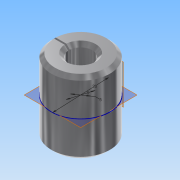
# Autodesk Inventor part: муфта
Saved by Autodesk Inventor 2017 (Build 210142000, 142)
## iProperties
Part Number: муфта
Material: Типовые
Document SubType Name: Modeling
Designer: Max
Density: 1 g/cm^3
Appearance: Алюминий — темный
Mass: 6.61019 g
Surface Area: 33.4899 cm^2
Volume: 6.61019 cm^3
Author: Max
Autodesk Inventor part; units mm, degrees
ref_plane "YZ Plane" through (0, 0, 0) normal (1, 0, 0) x (0, 1, 0)
ref_plane "XZ Plane" through (0, 0, 0) normal (0, 1, 0) x (-1, 0, 0)
ref_plane "XY Plane" through (0, 0, 0) normal (0, 0, 1) x (1, 0, 0)
sketch "Эскиз1" plane through (0, 0, 0) normal (0, 0, 1) x (1, 0, 0)
  circle A0 centre (0, 0) radius 10
  circle A1 centre (0, 0) radius 4
  circle A2 centre (0, 0) radius 2.5
  dimension "d0" = 20
  dimension "d1" = 8
  dimension "d2" = 5
  constraints: 3 centre point, 3 coincident
  measures "d0" diameter of A0
  measures "d1" diameter of A1
  measures "d2" diameter of A2
extrude "Выдавливание1" add sketch "Эскиз1" along normal blind 12.5 contours A0
extrude "Выдавливание2" add sketch "Эскиз1" against normal blind 12.5 contours A0 | A1
chamfer "Фаска1" distance 1.2 angle 45 4 edges at (-10, 0, -12.5) (-10, 0, 12.5) (-2.5, 0, -12.5) (-4, 0, 12.5)
sketch "Эскиз2" plane through (0, 0, -12.5) normal (0, 0, -1) x (-1, 0, 0)
  line L0 (10.8628, -0.3) -> (-0.9121, -0.3)
  line L1 (-0.9121, -0.3) -> (-0.9121, 0.3)
  line L2 (-0.9121, 0.3) -> (10.8628, 0.3)
  line L3 (10.8628, 0.3) -> (10.8628, -0.3)
  line L4 (10.8628, -0.3) -> (-0.9121, 0.3) construction
  line L5 (-0.9121, -0.3) -> (10.8628, 0.3) construction
  point P0 (0, 0)
  point P1 (4.9754, 0)
  dimension "d10" = 0.6
  dimension "d11" = 4.9754
  constraints: 12 end point, 2 midpoint, 2 parallel, 1 horizontal, 1 perpendicular
  measures "d10" distance between parallel lines of L0 L2
  measures "d11" distance of point (0, 0) point (4.975, 0)
extrude "Выдавливание3" cut sketch "Эскиз2" against normal blind 30
ref_plane "РабПлоскость1" through (0, 0, 0) normal (0, 0, -1) x (-1, 0, 0)
sketch "Эскиз3" plane through (0, 0, 0) normal (0, 0, -1) x (-1, 0, 0)
  circle A0 centre (0, 0) radius 10
  arc A1 (9.9955, 0.3) -> (9.9955, -0.3) centre (0, 0) ccw projected
  line L0 (-9.9999, -0.037) -> (9.9999, -0.037)
  constraints: 3 point on circle, 2 end point, 1 centre point, 1 coincident, 1 horizontal
extrude "Выдавливание4" cut sketch "Эскиз3" along normal mid plane 0.6 contours A0 L0 picked at (0.3426, 3.291)
sketch "Эскиз4" plane through (-8.7949, -0.3, -12.5) normal (0, 1, 0) x (1, 0, 0)
  circle A0 centre (1.7949, -6.25) radius 1.5
  circle A1 centre (1.7949, -18.75) radius 1.5
  line L0 (0, 0) -> (17.5949, 0) projected
  line L1 (17.5949, -25) -> (0, -25) projected
  point P0 (8.7949, -12.5)
  dimension "d17" = 3
  dimension "d18" = 3
  dimension "d19" = 6.25
  dimension "d20" = 6.25
  dimension "d21" = 7
  dimension "d22" = 7
  constraints: 2 centre point
  measures "d17" diameter of A0
  measures "d18" diameter of A1
  measures "d19" distance from line of L0 A0.centre
  measures "d20" distance from line of L1 A1.centre
  measures "d21" horizontal distance of point (8.795, -12.5) A0.centre
  measures "d22" horizontal distance of point (8.795, -12.5) A1.centre
extrude "Выдавливание5" cut sketch "Эскиз4" along normal blind 20
ref_plane "РабПлоскость2" through (-8.7949, 16.8, -12.5) normal (0, -1, 0) x (1, 0, 0)
sketch "Эскиз5" plane through (-8.7949, 16.8, -12.5) normal (0, -1, 0) x (1, 0, 0)
  spline S0 degree 4 poles (3.2949, 6.25) (3.2949, 5.9602) (3.2208, 5.6699) (3.0692, 5.4082) (2.6878, 5.0172) (2.4668, 4.8772) (2.2335, 4.7973) (1.7464, 4.728) (1.4956, 4.754) (1.2664, 4.8269) (0.9398, 5.0096) (0.8262, 5.0933) (0.7218, 5.1917) (0.5611, 5.39) (0.4993, 5.4829) (0.4449, 5.5852) (0.3514, 5.8208) (0.3144, 5.9563) (0.2949, 6.1031) (0.2949, 6.3424) (0.3027, 6.4345) (0.3175, 6.5243) (0.3688, 6.7319) (0.4112, 6.8451) (0.4631, 6.9492) (0.628, 7.2136) (0.7581, 7.3549) (0.9035, 7.4706) (1.203, 7.6372) (1.3518, 7.6953) (1.5105, 7.7323) (1.8327, 7.7576) (1.9958, 7.7485) (2.1612, 7.7149) (2.4707, 7.5983) (2.6146, 7.5207) (2.7487, 7.4198) (3.0679, 7.0941) (3.2204, 6.8318) (3.2949, 6.5407) (3.2949, 6.25) knots 0 0 0 0 0 0.110553 0.110553 0.110553 0.210117 0.210117 0.210117 0.323911 0.323911 0.323911 0.392633 0.392633 0.392633 0.443405 0.443405 0.443405 0.499546 0.499546 0.499546 0.534863 0.534863 0.534863 0.585287 0.585287 0.585287 0.6758 0.6758 0.6758 0.752528 0.752528 0.752528 0.824124 0.824124 0.824124 0.888854 0.888854 0.888854 1 1 1 1 1 projected
  spline S1 degree 4 poles (3.2949, 18.75) (3.2949, 18.4602) (3.2208, 18.1699) (3.0692, 17.9082) (2.6878, 17.5172) (2.4668, 17.3772) (2.2335, 17.2973) (1.7464, 17.228) (1.4956, 17.254) (1.2664, 17.3269) (0.9398, 17.5096) (0.8262, 17.5933) (0.7218, 17.6917) (0.5611, 17.89) (0.4993, 17.9829) (0.4449, 18.0852) (0.3514, 18.3208) (0.3144, 18.4563) (0.2949, 18.6031) (0.2949, 18.8424) (0.3027, 18.9345) (0.3175, 19.0243) (0.3688, 19.2319) (0.4112, 19.3451) (0.4631, 19.4492) (0.628, 19.7136) (0.7581, 19.8549) (0.9035, 19.9706) (1.203, 20.1372) (1.3518, 20.1953) (1.5105, 20.2323) (1.8327, 20.2576) (1.9958, 20.2485) (2.1612, 20.2149) (2.4707, 20.0983) (2.6146, 20.0207) (2.7487, 19.9198) (3.0679, 19.5941) (3.2204, 19.3318) (3.2949, 19.0407) (3.2949, 18.75) knots 0 0 0 0 0 0.110553 0.110553 0.110553 0.210117 0.210117 0.210117 0.323911 0.323911 0.323911 0.392633 0.392633 0.392633 0.443405 0.443405 0.443405 0.499546 0.499546 0.499546 0.534863 0.534863 0.534863 0.585287 0.585287 0.585287 0.6758 0.6758 0.6758 0.752528 0.752528 0.752528 0.824124 0.824124 0.824124 0.888854 0.888854 0.888854 1 1 1 1 1 projected
  circle A0 centre (1.7949, 6.25) radius 1.5 projected
  circle A1 centre (1.7949, 6.25) radius 2.25
  circle A2 centre (1.7949, 18.75) radius 1.5 projected
  circle A3 centre (1.7949, 18.75) radius 2.25
  point P0 (8.7949, 12.5)
  dimension "d26" = 4.5
  dimension "d27" = 4.5
  constraints: 2 centre point, 2 coincident, 2 horizontal alignment, 2 other
  measures "d26" diameter of A1
  measures "d27" diameter of A3
extrude "Выдавливание6" cut sketch "Эскиз5" along normal blind 14 contours S0 | S1 | A1 | A3
sketch "Эскиз6" plane through (-7, 2.8, -6.25) normal (0, 1, 0) x (1, 0, 0)
  circle A0 centre (0, 0) radius 1.5 projected
  circle A1 centre (0, 0) radius 2.25 projected
  circle A2 centre (0, -12.5) radius 1.5 projected
  circle A3 centre (0, -12.5) radius 2.25 projected
  circle A4 centre (0, 0) radius 2.1
  circle A5 centre (0, -12.5) radius 2.1
  point P0 (7, -6.25)
  dimension "d30" = 4.2
  dimension "d31" = 4.2
  constraints: 2 centre point, 2 coincident
  measures "d30" diameter of A4
  measures "d31" diameter of A5
extrude "Выдавливание7" add sketch "Эскиз6" along normal blind 4 contours A0 | A2 | A4 | A5
sketch "Эскиз7" plane through (-7, 6.8, -6.25) normal (0, 1, 0) x (1, 0, 0)
  line L0 (0, 1.1547) -> (1, 0.5774)
  line L1 (1, 0.5774) -> (1, -0.5774)
  line L2 (1, -0.5774) -> (0, -1.1547)
  line L3 (0, -1.1547) -> (-1, -0.5774)
  line L4 (-1, -0.5774) -> (-1, 0.5774)
  line L5 (-1, 0.5774) -> (0, 1.1547)
  circle A0 centre (0, -12.5) radius 2.25 projected
  line L6 (0, -11.3453) -> (1, -11.9226)
  line L7 (1, -11.9226) -> (1, -13.0774)
  line L8 (1, -13.0774) -> (0, -13.6547)
  line L9 (0, -13.6547) -> (-1, -13.0774)
  line L10 (-1, -13.0774) -> (-1, -11.9226)
  line L11 (-1, -11.9226) -> (0, -11.3453)
  point P0 (7, -6.25)
  point P1 (0, 0)
  dimension "d34" = 2
  dimension "d35" = 2
  constraints: 24 end point, 1 coincident, 26 other
  measures "d34" distance between parallel lines of L1 L4
  measures "d35" distance between parallel lines of L7 L10
extrude "Выдавливание8" cut sketch "Эскиз7" against normal blind 1.5 contours L0 L1 L2 L3 L4 L5 | L6 L7 L8 L9 L10 L11
fillet "Сопряжение1" radius 0.4 2 edges at (-9.1, 6.8, 6.25) (-9.1, 6.8, -6.25)
